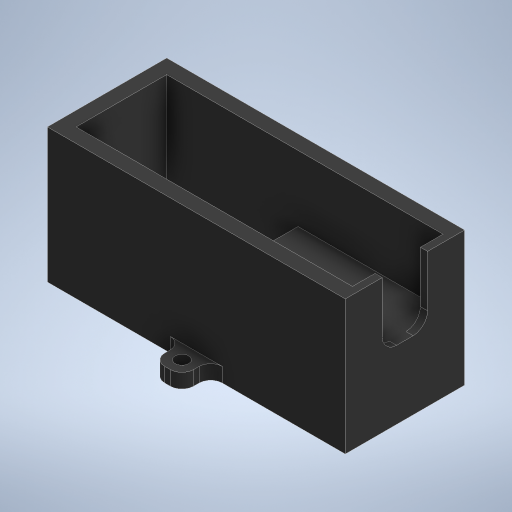
# Autodesk Inventor part: RadioMount
Saved by Autodesk Inventor 2024 (Build 280153000, 153)
## iProperties
Created: 2023-08-23
Part Number: RadioMount
Material: Rubber, Silicone
Document SubType Name: Modeling
Designer: 18179
Density: 1.25 g/cm^3
Appearance: Rubber - Black
Author: 18179
Autodesk Inventor part; units mm, degrees
ref_plane "YZ Plane" through (0, 0, 0) normal (1, 0, 0) x (0, 1, 0)
ref_plane "XZ Plane" through (0, 0, 0) normal (0, 1, 0) x (-1, 0, 0)
ref_plane "XY Plane" through (0, 0, 0) normal (0, 0, 1) x (1, 0, 0)
sketch "Sketch1" plane through (0, 0, 0) normal (0, 0, 1) x (1, 0, 0)
  line L0 (0, 0) -> (32, 0)
  line L1 (32, 0) -> (32, 11.938)
  line L2 (32, 11.938) -> (0, 11.938)
  line L3 (0, 11.938) -> (0, 0)
  line L4 (0, 0) -> (-29, 0)
  line L5 (-29, 0) -> (-29, 11.938)
  line L6 (-29, 11.938) -> (0, 11.938)
  line L7 (0, 11.938) -> (0, 0)
  line L8 (32, 11.938) -> (-9, 11.938)
  line L9 (-9, 11.938) -> (-9, 23.938)
  line L10 (-9, 23.938) -> (32, 23.938)
  line L11 (32, 23.938) -> (32, 11.938)
  line L12 (32, 0) -> (33.6002, 0)
  line L13 (33.6002, 0) -> (33.6002, 23.938)
  line L14 (33.6002, 23.938) -> (32, 23.938)
  line L15 (32, 23.938) -> (32, 0)
  line L16 (33.6002, 0) -> (-29, 0)
  line L17 (-29, 0) -> (-29, -3.175)
  line L18 (-29, -3.175) -> (33.6002, -3.175)
  line L19 (33.6002, -3.175) -> (33.6002, 0)
  line L20 (-29, -3.175) -> (-32.175, -3.175)
  line L21 (-32.175, -3.175) -> (-32.175, 23.938)
  line L22 (-32.175, 23.938) -> (-29, 23.938)
  line L23 (-29, 23.938) -> (-29, -3.175)
  line L24 (-32.175, 23.938) -> (33.6002, 23.938)
  line L25 (33.6002, 23.938) -> (33.6002, 27.113)
  line L26 (33.6002, 27.113) -> (-32.175, 27.113)
  line L27 (-32.175, 27.113) -> (-32.175, 23.938)
  dimension "d0" = 32
  dimension "d1" = 11.938
  dimension "d2" = 29
  dimension "d3" = 41
  dimension "d4" = 12
  dimension "d5" = 1.6002
  dimension "d7" = 3.175
  dimension "d8" = 3.175
  dimension "d9" = 3.175
  constraints: 56 end point, 14 parallel, 7 horizontal, 7 perpendicular, 2 collinear, 1 point on line
  measures "d0" distance of L2.end L1.end
  measures "d1" distance of L0.end L1.end
  measures "d2" distance of L5.end L6.end
  measures "d3" distance of L9.end L10.end
  measures "d4" distance of L8.end L9.end
  measures "d5" distance of L14.end L13.end
  measures "d7" distance of L18.end L12.end
  measures "d8" distance of L21.end L22.end
  measures "d9" distance of L25.end L24.end
extrude "Extrusion1" add sketch "Sketch1" along normal blind 20 contours L3 L2 L1 L0 | L0 L12 L19 L18 L17 L4 | L1 L11 L14 L13 L12 | L17 L20 L21 L22 L23 L5
sketch "Sketch2" plane through (0, 0, 20) normal (0, 0, 1) x (1, 0, 0)
  line L0 (-29, 23.938) -> (-32.175, 23.938) projected
  line L1 (-32.175, -3.175) -> (33.6002, -3.175) projected
  line L2 (-32.175, 23.938) -> (33.6002, 23.938)
  line L3 (33.6002, 23.938) -> (33.6002, -3.175)
  line L4 (33.6002, -3.175) -> (-32.175, -3.175)
  line L5 (-32.175, -3.175) -> (-32.175, 23.938)
  point P0 (0, 0)
  constraints: 8 end point, 2 parallel, 1 horizontal, 1 perpendicular
ref_plane "Work Plane1" through (0, 0, 10) normal (0, 0, 1) x (1, 0, 0)
extrude "Extrusion2" add sketch "Sketch2" along normal blind 3.175
mirror "Mirror1" about plane through (0, 0, 10) normal (0, 0, 1) of "Extrusion2"
sketch "Sketch3" plane through (33.6002, -3.175, 23.175) normal (1, 0, 0) x (0, 0, -1)
  line L0 (23.175, 15.113) -> (3.175, 15.113) projected
  line L1 (23.175, 27.113) -> (3.175, 27.113) projected
  line L2 (13.175, 15.113) -> (8.175, 15.113)
  line L3 (8.175, 15.113) -> (8.175, 27.113)
  line L4 (8.175, 27.113) -> (13.175, 27.113)
  line L5 (13.175, 27.113) -> (13.175, 15.113)
  line L6 (13.175, 27.113) -> (18.175, 27.113)
  line L7 (18.175, 27.113) -> (18.175, 15.113)
  line L8 (18.175, 15.113) -> (13.175, 15.113)
  line L9 (13.175, 15.113) -> (13.175, 27.113)
  point P0 (23.175, 3.175)
  dimension "d15" = 5
  dimension "d16" = 5
  constraints: 16 end point, 4 parallel, 2 horizontal, 2 perpendicular, 2 point on line, 1 midpoint
  measures "d15" distance of L3.end L4.end
  measures "d16" distance of L7.end L8.end
extrude "Extrusion3" cut sketch "Sketch3" against normal blind 3.175
fillet "Fillet1" radius 3.175 2 edges at (32.8001, 11.938, 5) (32.8001, 11.938, 15)
sketch "Sketch4" plane through (-32.175, -3.175, 23.175) normal (0, -1, 0) x (1, 0, 0)
  line L0 (65.7752, -8.175) -> (65.7752, 0) projected
  line L1 (65.7752, -26.35) -> (0, -26.35) projected
  line L2 (65.7752, 0) -> (0, 0)
  line L3 (0, 0) -> (0, -26.35)
  line L4 (0, -26.35) -> (65.7752, -26.35)
  line L5 (65.7752, -26.35) -> (65.7752, 0)
  line L6 (32.8876, 0) -> (36.0626, 0)
  line L7 (36.0626, 0) -> (36.0626, 6.35)
  line L8 (36.0626, 6.35) -> (32.8876, 6.35)
  line L9 (32.8876, 6.35) -> (32.8876, 0)
  line L10 (32.8876, 6.35) -> (29.7126, 6.35)
  line L11 (29.7126, 6.35) -> (29.7126, 0)
  line L12 (29.7126, 0) -> (32.8876, 0)
  line L13 (32.8876, 0) -> (32.8876, 6.35)
  circle A0 centre (32.8876, 3.175) radius 1.5
  line L14 (65.7752, -13.175) -> (55.6443, -13.175)
  line L15 (36.0626, -26.35) -> (36.0626, -32.7)
  line L16 (36.0626, -32.7) -> (32.8876, -32.7)
  line L17 (32.8876, -32.7) -> (29.7126, -32.7)
  line L18 (29.7126, -32.7) -> (29.7126, -26.35)
  circle A1 centre (32.8876, -29.525) radius 1.5
  point P0 (32.175, -23.175)
  dimension "d20" = 3.175
  dimension "d21" = 6.35
  dimension "d22" = 3.175
  dimension "d23" = 3
  constraints: 34 end point, 6 parallel, 6 symmetric about line, 4 horizontal, 3 midpoint, 3 perpendicular, 2 centre point, 1 point on line, 1 other
  measures "d20" distance of L8.end L7.end
  measures "d21" distance of L7.end L6.end
  measures "d22" distance of L12.end L11.end
  measures "d23" diameter of A0
extrude "Extrusion4" add sketch "Sketch4" against normal blind 3.175 contours L2 L9 A0 L8 L7 | L2 L11 L10 L9 A0 | L15 L16 L17 L18 L1
fillet "Fillet2" radius 2.54 8 edges at (-2.4624, -1.5875, 23.175) (-2.4624, -1.5875, 29.525) (3.8876, -1.5875, 29.525) (3.8876, -1.5875, 23.175) (-2.4624, -1.5875, -9.525) (3.8876, -1.5875, -9.525) (3.8876, -1.5875, -3.175) (-2.4624, -1.5875, -3.175)
sketch "Sketch5" plane through (-29, 23.938, 20) normal (0, 1, 0) x (1, 0, 0)
  line L0 (62.6002, 5) -> (61, 5) projected
  line L1 (61, 5) -> (61, 0) projected
  line L2 (61, 0) -> (0, 0) projected
  line L3 (0, 20) -> (0, 0) projected
  line L4 (61, 20) -> (0, 20) projected
  line L5 (61, 20) -> (61, 15) projected
  line L6 (61, 15) -> (62.6002, 15) projected
  line L7 (62.6002, 23.175) -> (62.6002, 15) projected
  line L8 (62.6002, 23.175) -> (-3.175, 23.175) projected
  line L9 (-3.175, 23.175) -> (-3.175, -3.175) projected
  line L10 (62.6002, -3.175) -> (-3.175, -3.175) projected
  line L11 (62.6002, 5) -> (62.6002, -3.175) projected
  point P0 (29, 20)
extrude "Extrusion5" add sketch "Sketch5" along normal blind 2.54
body "Solid1"
